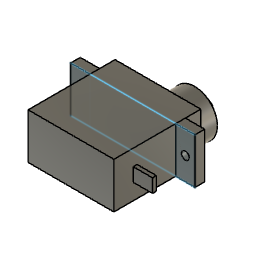
SG90 v2 (Autodesk Fusion 360 design; units mm, degrees)
Autodesk Fusion 360 part; units mm, degrees
sketch "Sketch1" plane through (0, 0, 0) normal (0, 0, 1) x (1, 0, 0)
  line L0 (0, 0) -> (22.2, 0)
  line L1 (22.2, 0) -> (22.2, 16)
  line L2 (22.2, 16) -> (0, 16)
  line L3 (0, 16) -> (0, 0)
  dimension "d1" = 22.2
  constraint horizontal L0
  constraint vertical L1
  constraint horizontal L2
  constraint vertical L3
  constraint coincident L0.start L3.end
  measures "d1" distance of L1.end L2.end
extrude "Extrude1" add sketch "Sketch1" along normal blind 11.8 makes body 1
sketch "Sketch2" plane through (0, 16, 0) normal (0, 1, 0) x (-1, 0, 0)
  line L0 (-22.2, 0) -> (0, 0)
  line L1 (0, 0) -> (0, 11.8)
  line L2 (0, 11.8) -> (-22.2, 11.8)
  line L3 (-22.2, 11.8) -> (-22.2, 0)
  line L4 (-27.2, 0) -> (5, 0)
  line L5 (5, 0) -> (5, 11.8)
  line L6 (5, 11.8) -> (-27.2, 11.8)
  line L7 (-27.2, 11.8) -> (-27.2, 0)
  dimension "d4" = 32.2
  dimension "d5" = 5
  constraint horizontal L4
  constraint vertical L5
  constraint horizontal L6
  constraint vertical L7
  measures "d4" distance of L4.start L4.end
  measures "d5" distance of L1 L5
extrude "Extrude3" add sketch "Sketch2" along normal blind 6.5 contours L0 L1 L2 L3 L4 L6 bodies 1
extrude "Extrude2" add sketch "Sketch2" along normal blind 2.5 separate body contours L3 L4 L6 L7 | L1 L4 L5 L6 makes body 2 at (23.8667, 16, 3.9333) makes body 3 at (-3.3333, 16, 7.8667)
sketch "Sketch4" plane through (0, 22.5, 0) normal (0, 1, 0) x (-1, 0, 0)
  line L0 (0, 0) -> (0, 11.8)
  line L1 (0, 11.8) -> (-22.2, 11.8)
  line L2 (-22.2, 11.8) -> (-22.2, 0)
  line L3 (-22.2, 0) -> (0, 0)
  circle A0 centre (-16.3, 5.9) radius 5.9
  line L4 (5, 11.8) -> (-27.2, 11.8)
  dimension "d13" = 5.9
  dimension "d14" = 5.9
  dimension "d15" = 11.8
  measures "d13" distance of A0.centre L4
  measures "d14" distance of L2 A0.centre
  measures "d15" diameter of A0
extrude "Extrude5" add sketch "Sketch4" along normal blind 4.3 contours A0 bodies 1
sketch "Sketch5" plane through (0, 26.8, 0) normal (0, 1, 0) x (-1, 0, 0)
  circle A0 centre (-16.3, 5.9) radius 5.9
  circle A1 centre (-16.3, 5.9) radius 2.25
  dimension "d18" = 4.5
  constraint concentric A0 A1
  measures "d18" diameter of A1
extrude "Extrude6" add sketch "Sketch5" along normal blind 2.7 contours A1 bodies 1
sketch "Sketch6" plane through (22.2, 0, 0) normal (1, 0, 0) x (0, 1, 0)
  line L0 (0, 0) -> (22.5, 0)
  line L1 (22.5, 0) -> (22.5, 5.9)
  line L2 (22.5, 5.9) -> (22.5, 11.8)
  line L3 (22.5, 11.8) -> (0, 11.8)
  line L4 (0, 11.8) -> (0, 0)
  line L5 (5, 7.65) -> (6, 7.65)
  line L6 (6, 7.65) -> (6, 4.15)
  line L7 (6, 4.15) -> (5, 4.15)
  line L8 (5, 4.15) -> (5, 7.65)
  dimension "d21" = 3.5
  dimension "d22" = 1
  dimension "d23" = 4.15
  constraint horizontal L5
  constraint vertical L6
  constraint horizontal L7
  constraint vertical L8
  measures "d21" distance of L5.end L6.end
  measures "d22" distance of L5.start L5.end
  measures "d23" distance of L0 L7
extrude "Extrude7" add sketch "Sketch6" along normal blind 5 contours L5 L6 L7 L8 bodies 1
sketch "Sketch7" plane through (0, 18.5, 0) normal (0, 1, 0) x (-1, 0, 0)
  line L0 (-22.2, 11.8) -> (-27.2, 11.8)
  line L1 (-27.2, 11.8) -> (-27.2, 0)
  line L2 (-27.2, 0) -> (-22.2, 0)
  line L3 (-22.2, 0) -> (-22.2, 11.8)
  circle A0 centre (-24.7, 5.9) radius 1
  circle A1 centre (2.5, 5.9) radius 1
  line L4 (5, 11.8) -> (-27.2, 11.8)
  line L5 (5, 0) -> (5, 11.8)
  dimension "d26" = 27.2
  dimension "d27" = 2
  dimension "d28" = 2
  dimension "d29" = 5.9
  dimension "d30" = 2.5
  measures "d26" distance of A0.centre A1.centre
  measures "d27" diameter of A0
  measures "d28" diameter of A1
  measures "d29" distance of A1.centre L4
  measures "d30" distance of A1.centre L5
extrude "Extrude8" cut sketch "Sketch7" against normal blind 2.5 contours A0 | A1 bodies 2 3
equation "d16 = 6 mm - 1.7 mm"
equation "d19 = 3.00 mm - 0.3 mm"
